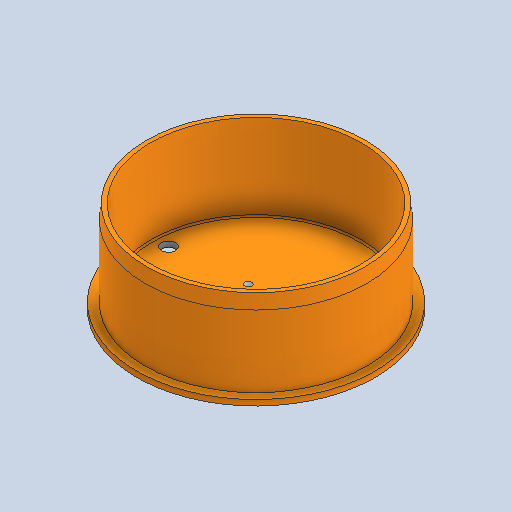
# Autodesk Inventor part: Cap_pipes
Saved by Autodesk Inventor 2023.1 (Build 271208000, 208)
## iProperties
Created: 2023-12-24
Part Number: Cap_pipes
Material: Типовые
Document SubType Name: Modeling
Designer: Dell
Density: 1 g/cm^3
Appearance: По умолчанию
Author: Dell
Autodesk Inventor part; units mm, degrees
ref_plane "YZ Plane" through (0, 0, 0) normal (1, 0, 0) x (0, 1, 0)
ref_plane "XZ Plane" through (0, 0, 0) normal (0, 1, 0) x (-1, 0, 0)
ref_plane "XY Plane" through (0, 0, 0) normal (0, 0, 1) x (1, 0, 0)
sketch "Эскиз2" plane through (0, 0, 0) normal (1, 0, 0) x (0, 1, 0)
  line L0 (0, 16.9979) -> (0, -102.0021) projected
  line L1 (18.2354, -0.0021) -> (-21.7975, -0.0021) construction
  line L2 (0, -85.0021) -> (4, -85.0021)
  line L3 (4, -85.0021) -> (4, -79.0021)
  line L4 (4, -75.0021) -> (65, -75.0021)
  line L5 (65, -75.0021) -> (65, -78.0021)
  line L6 (65, -79.0021) -> (65, -75.0021) construction
  line L7 (4, -79.0021) -> (55, -79.0021)
  line L8 (55, -79.0021) -> (65, -78.0021)
  line L9 (4, -75.0021) -> (4, -4.0021)
  line L10 (0, -85.0021) -> (0, -4.0021)
  line L11 (0, -4.0021) -> (4, -4.0021)
  point P0 (0, -0.0021)
  point P1 (4, -0.0021)
  dimension "d1" = 4
  dimension "d2" = 6
  dimension "d3" = 61
  dimension "d6" = 3
  dimension "d7" = 51
  dimension "d8" = 4
  constraints: 22 end point, 4 horizontal, 4 point on line, 3 vertical, 2 perpendicular
  measures "d1" distance of L2.start L2.end
  measures "d2" distance of L2.end L3.end
  measures "d3" distance of L3.end L6.start
  measures "d6" distance of L4.end L5.end
  measures "d7" distance of L3.end L7.end
  measures "d8" distance between parallel lines of L4 L7
revolve "Вращение1" add sketch "Эскиз2" angle 360 about axis through (0, 18.2354, -0.0021) along (0, -1, 0)
fillet "Сопряжение1" radius 1 1 edges at (0, 4, 74.9979)
sketch "Эскиз3" plane through (0, 4, -0.0021) normal (0, 1, 0) x (1, 0, 0)
  ellipse E0 centre (-13.967, 8.3729) end of major axis (-13.9806, 5.1229) minor radius 3.25 construction
  circle A0 centre (13.8163, -8.069) radius 3.25 construction
  circle A1 centre (13.8163, -8.069) radius 2.5 projected
  circle A2 centre (-13.967, 8.3729) radius 2.5 projected
  arc A3 (-64.2334, 5.859) -> (-62.6955, 4.3359) centre (-65.4333, 3.1094) ccw projected
  circle A4 centre (-65.4333, 3.1094) radius 5
  point P0 (0, -0.0021)
  dimension "d14" = 10
  constraints: 1 centre point, 1 coincident, 1 other
  measures "d14" diameter of A4
extrude "Выдавливание1" cut sketch "Эскиз3" against normal blind 10
